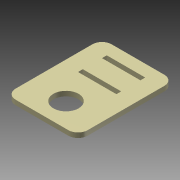
# Autodesk Inventor part: 26051-01
Saved by Autodesk Inventor 2014 (Build 180170000, 170)
## iProperties
Category: stocked
Created: 2013-05-31
Part Number: 26051-01
Material: Nylon 6/6
Document SubType Name: Modeling
Designer: Edward
Density: 1.13 g/cm^3
Stock Number: B17065
Mass: 0.292578 g
Surface Area: 6.36897 cm^2
Volume: 0.258919 cm^3
Description: fiberglass in-line belt clip
Vendor: custom
Project: Shapeoko
Appearance: Nylon 6
User Status: W
Authority: PER WOODY @ INVISIBLE LIGHT 9-16-13
Author: Edward
Subject: Clamping
Comments: Fusion
Title: Fiberglass Belt Clip
Autodesk Inventor part; units mm, degrees
ref_plane "YZ Plane" through (0, 0, 0) normal (1, 0, 0) x (0, 1, 0)
ref_plane "XZ Plane" through (0, 0, 0) normal (0, 1, 0) x (-1, 0, 0)
ref_plane "XY Plane" through (0, 0, 0) normal (0, 0, 1) x (1, 0, 0)
sketch "Sketch1" plane through (0, 0, 0) normal (0, 0, 1) x (1, 0, 0)
  line L0 (-7.5, 10) -> (7.5, 10)
  line L1 (7.5, 10) -> (7.5, -10)
  line L2 (7.5, -10) -> (-7.5, -10)
  line L3 (-7.5, -10) -> (-7.5, 10)
  point P0 (0, 0)
  dimension "d0" = 15
  dimension "d1" = 20
  dimension "d2" = 7.5
  dimension "d3" = 10
  constraints: 8 end point, 2 parallel, 1 horizontal, 1 perpendicular
  measures "d0" distance of L1.end L2.end
  measures "d1" distance of L0.end L1.end
  measures "d2" distance from line of point (0, 0) L3
  measures "d3" distance from line of L0 point (0, 0)
extrude "Extrusion1" add sketch "Sketch1" along normal blind 1
fillet "Fillet1" radius 2 4 edges at (7.5, 10, 0.5) (-7.5, 10, 0.5) (7.5, -10, 0.5) (-7.5, -10, 0.5)
sketch "Sketch2" plane through (0, 0, 1) normal (0, 0, 1) x (1, 0, 0)
  line L0 (-5.5, -10) -> (5.5, -10) projected
  line L1 (5.5, 10) -> (-5.5, 10) projected
  line L2 (-7.5, 8) -> (-7.5, -8) projected
  line L3 (-4, 7.5) -> (4, 7.5)
  line L4 (4, 7.5) -> (4, 6.5)
  line L5 (4, 6.5) -> (-4, 6.5)
  line L6 (-4, 6.5) -> (-4, 7.5)
  line L7 (-4, 2.5) -> (4, 2.5)
  line L8 (4, 2.5) -> (4, 1.5)
  line L9 (4, 1.5) -> (-4, 1.5)
  line L10 (-4, 1.5) -> (-4, 2.5)
  circle A0 centre (0, -5) radius 2.625
  point P0 (0, 0)
  dimension "d7" = 8
  dimension "d8" = 1
  dimension "d9" = 3.5
  dimension "d10" = 2.5
  dimension "d11" = 1
  dimension "d12" = 4
  dimension "d13" = 3.5
  dimension "d14" = 8
  dimension "d15" = 5.25
  dimension "d16" = 5
  dimension "d17" = 7.5
  constraints: 16 end point, 4 parallel, 2 horizontal, 2 perpendicular, 1 centre point
  measures "d7" distance of L4.end L5.end
  measures "d8" distance of L3.end L4.end
  measures "d9" distance between parallel lines of L2 L6
  measures "d10" distance between parallel lines of L1 L3
  measures "d11" distance of L7.end L8.end
  measures "d12" distance between parallel lines of L5 L7
  measures "d13" distance between parallel lines of L2 L10
  measures "d14" distance of L7.start L7.end
  measures "d15" diameter of A0
  measures "d16" distance from line of L0 A0.centre
  measures "d17" distance from line of L2 A0.centre
extrude "Extrusion2" cut sketch "Sketch2" against normal through all
equation "\"d2\" = 0.5 * d0"
equation "\"d3\" = 0.5 * d1"
body "Solid1"
